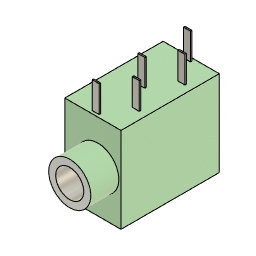
Headphone amplifier II v17 (Autodesk Fusion 360 archive; units mm, degrees)
design "Jack"
Autodesk Fusion 360 part; units mm, degrees
sketch "Sketch1" plane through (0, 0, 0) normal (0, 0, 1) x (1, 0, 0)
  line L0 (4, -7) -> (-4, -7)
  line L1 (-4, -7) -> (-4, 7)
  line L2 (-4, 7) -> (4, 7)
  line L3 (4, 7) -> (4, -7)
  line L4 (4, -7) -> (-4, 7) construction
  line L5 (-4, -7) -> (4, 7) construction
  line L6 (0.5, -0.1) -> (-0.5, -0.1)
  line L7 (-0.5, -0.1) -> (-0.5, 0.1)
  line L8 (-0.5, 0.1) -> (0.5, 0.1)
  line L9 (0.5, 0.1) -> (0.5, -0.1)
  line L10 (0.5, -0.1) -> (-0.5, 0.1) construction
  line L11 (-0.5, -0.1) -> (0.5, 0.1) construction
  line L12 (0.5, -6.6) -> (-0.5, -6.6)
  line L13 (-0.5, -6.6) -> (-0.5, -6.4)
  line L14 (0.5, -6.4) -> (0.5, -6.6)
  line L15 (-0.5, -6.4) -> (0.5, -6.4)
  line L16 (2.959, -3.35) -> (1.959, -3.35)
  line L17 (1.959, -3.35) -> (1.959, -3.15)
  line L18 (2.959, -3.15) -> (2.959, -3.35)
  line L19 (1.959, -3.15) -> (2.959, -3.15)
  line L20 (2.959, 3.15) -> (1.959, 3.15)
  line L21 (1.959, 3.15) -> (1.959, 3.35)
  line L22 (2.959, 3.35) -> (2.959, 3.15)
  line L23 (1.959, 3.35) -> (2.959, 3.35)
  line L24 (0.5, 6.4) -> (-0.5, 6.4)
  line L25 (-0.5, 6.4) -> (-0.5, 6.6)
  line L26 (0.5, 6.6) -> (0.5, 6.4)
  line L27 (-0.5, 6.6) -> (0.5, 6.6)
  dimension "d61" = 8
  dimension "d62" = 14
  dimension "d63" = 1
  dimension "d64" = 0.2
  dimension "d67" = 2.459
  dimension "d68" = 6.5
  constraint horizontal L0
  constraint perpendicular L0 L1
  constraint parallel L0 L2
  constraint parallel L1 L3
  constraint coincident L4 origin
  constraint coincident L5 origin
  constraint horizontal L6
  constraint perpendicular L6 L7
  constraint parallel L6 L8
  constraint parallel L7 L9
  constraint coincident L10 origin
  constraint coincident L11 origin
  measures "d61" distance of L1.end L2.end
  measures "d62" distance of L0.end L1.end
  measures "d63" distance of L7.end L8.end
  measures "d64" distance of L6.end L7.end
extrude "Extrude1" add sketch "Sketch1" along normal blind 16 contours L6 L7 L8 L9 | L12 L13 L14 L15 | L16 L17 L18 L19 | L20 L21 L22 L23 | L24 L25 L26 L27 makes body 1 at (0.1667, -0.1, 5.3333) makes body 2 at (2.6257, 3.15, 5.3333) makes body 3 at (2.6257, -3.35, 5.3333) makes body 4 at (0.1667, 6.4, 5.3333) makes body 5 at (0.1667, -6.6, 5.3333)
extrude "Extrude2" add sketch "Sketch1" along normal blind 12.2 bodies 1 2 3 4 5
sketch "Sketch2" plane through (0, -7, 0) normal (0, -1, 0) x (1, 0, 0)
  line L0 (-4, 0) -> (4, 0)
  line L1 (4, 0) -> (4, 12.2)
  line L2 (4, 12.2) -> (-4, 12.2)
  line L3 (-4, 12.2) -> (-4, 0)
  circle A0 centre (0.7, 6) radius 3
  circle A1 centre (0.7, 6) radius 2
  line L4 (4, 0) -> (-4, 0)
  dimension "d73" = 6
  dimension "d74" = -1
  dimension "d76" = 3.3
  dimension "d78" = 6
  measures "d73" diameter of A0
  measures "d76" distance of L1 A0.centre
  measures "d78" distance of A0.centre L4
extrude "Extrude3" add sketch "Sketch2" along normal blind 4 contours A0 bodies 1
extrude "Extrude4" cut sketch "Sketch2" against normal blind 12 contours A1 bodies 1
named bodies: "JackFem"

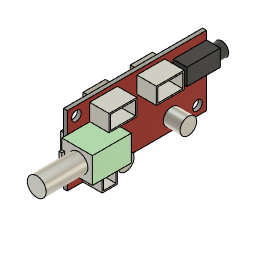
design "Amplifier"
Autodesk Fusion 360 part; units mm, degrees
sketch "Sketch1" plane through (0, 0, 0) normal (0, 0, 1) x (1, 0, 0)
  line L0 (12.5, -25) -> (-12.5, -25)
  line L1 (-12.5, -25) -> (-12.5, 25)
  line L2 (-12.5, 25) -> (12.5, 25)
  line L3 (12.5, 25) -> (12.5, -25)
  line L4 (12.5, -25) -> (-12.5, 25) construction
  line L5 (-12.5, -25) -> (12.5, 25) construction
  circle A0 centre (9.25, 21.75) radius 1.75
  circle A1 centre (-9.25, -21.75) radius 1.75
  line L6 (4.3, -27) -> (-5, -27)
  line L7 (-5, -27) -> (-5, -13)
  line L8 (-5, -13) -> (4.3, -13)
  line L9 (4.3, -13) -> (4.3, -27)
  line L10 (4.3, -27) -> (-5, -13) construction
  line L11 (-5, -27) -> (4.3, -13) construction
  line L12 (-3.5, 13) -> (-9.5, 13)
  line L13 (-9.5, 13) -> (-9.5, 25)
  line L14 (-9.5, 25) -> (-3.5, 25)
  line L15 (-3.5, 25) -> (-3.5, 13)
  line L16 (-3.5, 13) -> (-9.5, 25) construction
  line L17 (-9.5, 13) -> (-3.5, 25) construction
  line L18 (-11.1, -7) -> (-5.1, -7)
  line L19 (-5.1, -7) -> (-5.1, -17)
  line L20 (-5.1, -17) -> (-11.1, -17)
  line L21 (-11.1, -17) -> (-11.1, -7)
  line L22 (-11.1, -7) -> (-5.1, -17) construction
  line L23 (-5.1, -7) -> (-11.1, -17) construction
  line L24 (-10.6, -7.5) -> (-5.6, -7.5)
  line L25 (-5.6, -7.5) -> (-5.6, -16.5)
  line L26 (-5.6, -16.5) -> (-10.6, -16.5)
  line L27 (-10.6, -16.5) -> (-10.6, -7.5)
  line L28 (-11.1, 0) -> (-11.1, 10)
  line L29 (-11.1, 10) -> (-5.1, 10)
  line L30 (-5.1, 10) -> (-5.1, 0)
  line L31 (-5.1, 0) -> (-11.1, 0)
  line L32 (-10.6, 0.5) -> (-10.6, 9.5)
  line L33 (-10.6, 9.5) -> (-5.6, 9.5)
  line L34 (-5.6, 0.5) -> (-10.6, 0.5)
  line L35 (-5.6, 9.5) -> (-5.6, 0.5)
  circle A2 centre (8, 12.5) radius 3
  circle A3 centre (8, -10) radius 3
  line L36 (4.4, -14) -> (12.4, -14)
  line L37 (12.4, -14) -> (12.4, -19.5)
  line L38 (12.4, -19.5) -> (4.4, -19.5)
  line L39 (4.4, -19.5) -> (4.4, -14)
  line L40 (4.4, -14) -> (12.4, -19.5) construction
  line L41 (12.4, -14) -> (4.4, -19.5) construction
  line L42 (4.9, -14.5) -> (11.9, -14.5)
  line L43 (11.9, -14.5) -> (11.9, -19)
  line L44 (11.9, -19) -> (4.9, -19)
  line L45 (4.9, -19) -> (4.9, -14.5)
  point P0 (-0.35, -20)
  point P1 (-6.5, 19)
  point P2 (-8.1, -12)
  point P3 (8.4, -16.75)
  dimension "d1" = 25
  dimension "d2" = 50
  dimension "d3" = 3.5
  dimension "d4" = 3.25
  dimension "d5" = 3.25
  dimension "d6" = 3.25
  dimension "d7" = 3.25
  dimension "d8" = 9.3
  dimension "d9" = 14
  dimension "d10" = 7.5
  dimension "d11" = 2
  dimension "d12" = 12
  dimension "d13" = 6
  dimension "d15" = 3
  dimension "d30" = 6
  dimension "d31" = 10
  dimension "d32" = 0.5
  dimension "d33" = 0.5
  dimension "d34" = 6
  dimension "d35" = 10
  dimension "d37" = 8
  dimension "d38" = 7
  dimension "d39" = 1.4
  dimension "d40" = 6
  dimension "d41" = 12.5
  dimension "d42" = 35
  dimension "d43" = 4.5
  dimension "d44" = 8
  dimension "d45" = 5.5
  dimension "d46" = 0.5
  dimension "d47" = 0.1
  dimension "d48" = 5.5
  constraint horizontal L0
  constraint perpendicular L0 L1
  constraint parallel L0 L2
  constraint parallel L1 L3
  constraint coincident L4 origin
  constraint coincident L5 origin
  constraint equal A0 A1
  constraint horizontal L6
  constraint perpendicular L6 L7
  constraint parallel L6 L8
  constraint parallel L7 L9
  constraint coincident L10 P0
  constraint coincident L11 P0
  constraint horizontal L12
  constraint perpendicular L12 L13
  constraint parallel L12 L14
  constraint parallel L13 L15
  constraint coincident L16 P1
  constraint coincident L17 P1
  constraint horizontal L18
  constraint perpendicular L18 L19
  constraint parallel L18 L20
  constraint parallel L19 L21
  constraint coincident L22 P2
  constraint coincident L23 P2
  constraint horizontal L29
  constraint perpendicular L29 L30
  constraint parallel L29 L31
  constraint parallel L28 L30
  constraint vertical L18.end L30.end
  constraint equal A2 A3
  constraint vertical A2.centre A3.centre
  constraint horizontal L36
  constraint perpendicular L36 L37
  constraint parallel L36 L38
  constraint parallel L37 L39
  constraint coincident L40 P3
  constraint coincident L41 P3
  constraint coincident L2 L13.end
  measures "d1" distance of L1.end L2.end
  measures "d2" distance of L0.end L1.end
  measures "d3" diameter of A0
  measures "d4" distance of L2 A0.centre
  measures "d5" distance of L3 A0.centre
  measures "d6" distance of L1 A1.centre
  measures "d7" distance of L0 A1.centre
  measures "d8" distance of L7.end L8.end
  measures "d9" distance of L6.end L7.end
  measures "d10" distance of L1 L7
  measures "d11" distance of L0 L6
  measures "d12" distance of L12.start L14.end
  measures "d13" distance of L12.start L12.end
  measures "d15" distance of L1 L13
  measures "d30" distance of L19.end L20.end
  measures "d31" distance of L18.end L19.end
  measures "d34" distance of L30.end L28.start
  measures "d35" distance of L29.end L30.end
  measures "d37" distance of L0 L20
  measures "d38" distance of L18 L31
  measures "d39" distance of L1 L21
  measures "d40" diameter of A2
  measures "d41" distance of L2 A2.centre
  measures "d42" distance of L2 A3.centre
  measures "d43" distance of L3 A2.centre
  measures "d44" distance of L37.end L38.end
  measures "d45" distance of L36.end L37.end
  measures "d47" distance of L3 L37
  measures "d48" distance of L0 L38
extrude "Extrude1" add sketch "Sketch1" against normal blind 1.4 contours L0 L1 L2 L3 L7 L8 L9 L12 L13 L15 | L0 L7 L8 L9 | L2 L12 L13 L14 L15 | L18 L19 L20 L21 | L24 L25 L26 L27 | L28 L29 L30 L31 | L32 L33 L34 L35 | A2 | A3 | L36 L37 L38 L39 | L42 L43 L44 L45
sketch "Sketch5" plane through (0, 0, -1.4) normal (0, 0, -1) x (1, 0, 0)
  circle A0 centre (9.25, -21.75) radius 1.75
  circle A1 centre (-9.25, 21.75) radius 1.75
  line L0 (-12.5, -25) -> (12.5, -25)
  line L1 (12.5, -25) -> (12.5, 25)
  line L2 (12.5, 25) -> (-12.5, 25)
  line L3 (-12.5, 25) -> (-12.5, -25)
  line L4 (-7, 8) -> (-12, 8)
  line L5 (-12, 8) -> (-12, 16)
  line L6 (-12, 16) -> (-7, 16)
  line L7 (-7, 16) -> (-7, 8)
  line L8 (-7, 8) -> (-12, 16) construction
  line L9 (-12, 8) -> (-7, 16) construction
  line L10 (-7, -1) -> (-7, -9)
  line L11 (-7, -9) -> (-12, -9)
  line L12 (-12, -9) -> (-12, -1)
  line L13 (-12, -1) -> (-7, -1)
  line L14 (4, 19) -> (-4, 19)
  line L15 (-4, 19) -> (-4, 24)
  line L16 (-4, 24) -> (4, 24)
  line L17 (4, 24) -> (4, 19)
  line L18 (4, 12) -> (-4, 12)
  line L19 (-4, 12) -> (-4, 17)
  line L20 (-4, 17) -> (4, 17)
  line L21 (4, 17) -> (4, 12)
  line L22 (11.5, 17) -> (5.5, 17)
  line L23 (5.5, 17) -> (5.5, 20)
  line L24 (5.5, 20) -> (11.5, 20)
  line L25 (11.5, 20) -> (11.5, 17)
  line L26 (11.5, 17) -> (5.5, 20) construction
  line L27 (5.5, 17) -> (11.5, 20) construction
  line L28 (4, 24) -> (-4, 19) construction
  line L29 (-4, 24) -> (4, 19) construction
  point P0 (-9.5, 12)
  point P1 (8.5, 18.5)
  point P2 (0, 21.5)
  dimension "d100" = 5
  dimension "d101" = 8
  dimension "d104" = 5
  dimension "d105" = 8
  dimension "d106" = 5
  dimension "d107" = 8
  dimension "d108" = 5
  dimension "d109" = 8
  dimension "d110" = 6
  dimension "d111" = 3
  dimension "d112" = 13
  dimension "d113" = 26
  dimension "d114" = 3
  dimension "d115" = 12.5
  dimension "d116" = 1
  dimension "d117" = 8
  dimension "d118" = 5
  dimension "d119" = 1
  constraint horizontal L4
  constraint perpendicular L4 L5
  constraint parallel L4 L6
  constraint parallel L5 L7
  constraint coincident L8 P0
  constraint coincident L9 P0
  constraint horizontal L11
  constraint perpendicular L11 L12
  constraint parallel L11 L13
  constraint parallel L10 L12
  constraint perpendicular L15 L16
  constraint parallel L15 L17
  constraint parallel L14 L16
  constraint perpendicular L19 L20
  constraint parallel L19 L21
  constraint parallel L18 L20
  constraint horizontal L22
  constraint perpendicular L22 L23
  constraint parallel L22 L24
  constraint parallel L23 L25
  constraint coincident L26 P1
  constraint coincident L27 P1
  constraint vertical L4.end L12.end
  constraint vertical L14.end L19.end
  constraint parallel L17 L21
  constraint midpoint L28 P2
  measures "d100" distance of L5.end L6.end
  measures "d101" distance of L4.end L5.end
  measures "d104" distance of L12.end L10.start
  measures "d105" distance of L12.end L11.end
  measures "d106" distance of L16.end L14.start
  measures "d107" distance of L16.end L15.end
  measures "d108" distance of L20.end L18.start
  measures "d109" distance of L20.end L19.end
  measures "d110" distance of L23.end L24.end
  measures "d111" distance of L22.end L23.end
  measures "d112" distance of L2 P0
  measures "d113" distance of L2 L13
  measures "d114" distance of L3 P0
  measures "d115" distance of L3 P2
  measures "d116" distance of L2 L16
  measures "d117" distance of L2 L20
  measures "d118" distance of L2 L24
  measures "d119" distance of L1 L25
extrude "Extrude11" add sketch "Sketch5" along normal blind 2 contours L4 L5 L6 L7 | L10 L11 L12 L13 | L14 L15 L16 L17 | L18 L19 L20 L21 | L22 L23 L24 L25
extrude "Extrude2" add sketch "Sketch1" along normal blind 5 contours L2 L12 L13 L14 L15
extrude "Extrude10" add sketch "Sketch1" along normal blind 7 contours L36 L37 L38 L39
sketch "Sketch3" plane through (0, 25, 0) normal (0, 1, 0) x (-1, 0, 0)
  line L0 (12.5, 0) -> (9.5, 0)
  line L1 (9.5, 0) -> (9.5, 5)
  line L2 (9.5, 5) -> (3.5, 5)
  line L3 (3.5, 5) -> (3.5, 0)
  line L4 (3.5, 0) -> (-12.5, 0)
  line L5 (-12.5, 0) -> (-12.5, -1.4)
  line L6 (-12.5, -1.4) -> (12.5, -1.4)
  line L7 (12.5, -1.4) -> (12.5, 0)
sketch "Sketch4" plane through (0, 25, 1.8) normal (0, 1, 0) x (-1, 0, 0)
  line L0 (9.5, 3.2) -> (3.5, 3.2)
  line L1 (3.5, 3.2) -> (3.5, -1.8)
  circle A0 centre (6.5, 0.7) radius 2.5
  circle A1 centre (6.5, 0.7) radius 2
  point P0 (6.5, 3.2)
  point P1 (3.5, 0.7)
  dimension "d53" = 5
  dimension "d54" = -0.5
  constraint midpoint L0 P0
  constraint midpoint L1 P1
  constraint vertical P0 A0.centre
  constraint horizontal P1 A0.centre
  measures "d53" diameter of A0
extrude "Extrude8" add sketch "Sketch4" along normal blind 3
extrude "Extrude9" cut sketch "Sketch4" against normal blind 10 contours A1
extrude "Extrude3" add sketch "Sketch1" along normal blind 11 contours L0 L6 L7 L9 | L0 L7 L8 L9
sketch "Sketch2" plane through (0, -27, 0) normal (0, -1, 0) x (1, 0, 0)
  line L0 (-5, 0) -> (4.3, 0)
  line L1 (4.3, 0) -> (4.3, 11)
  line L2 (4.3, 11) -> (-5, 11)
  line L3 (-5, 11) -> (-5, 0)
  circle A0 centre (-0.35, 6) radius 3.4
  line L4 (0.65, 0) -> (-1.35, 0)
  line L5 (-1.35, 0) -> (-1.35, 1)
  line L6 (-1.35, 1) -> (0.65, 1)
  line L7 (0.65, 1) -> (0.65, 0)
  line L8 (0.65, 0) -> (-1.35, 1) construction
  line L9 (-1.35, 0) -> (0.65, 1) construction
  point P0 (-0.35, 11)
  point P1 (-0.35, 0.5)
  point P2 (-0.35, 0)
  dimension "d22" = 6.8
  dimension "d23" = 5
  dimension "d26" = 2
  dimension "d27" = 1
  constraint midpoint L2 P0
  constraint vertical A0.centre P0
  constraint horizontal L4
  constraint perpendicular L4 L5
  constraint parallel L4 L6
  constraint parallel L5 L7
  constraint coincident L8 P1
  constraint coincident L9 P1
  constraint vertical A0.centre P1
  constraint coincident L4 P2
  measures "d22" diameter of A0
  measures "d23" distance of L2 A0.centre
  measures "d26" distance of L5.end L6.end
  measures "d27" distance of L4.end L5.end
extrude "Extrude4" add sketch "Sketch2" along normal blind 15 contours A0
extrude "Extrude5" add sketch "Sketch2" along normal blind 1 contours L0 L4 L5 L6 L7
extrude "Extrude6" add sketch "Sketch1" along normal blind 6 contours A2 | A3
extrude "Extrude7" add sketch "Sketch1" along normal blind 7 contours L18 L19 L20 L21 | L28 L29 L30 L31
move_body "Move1" bodies 1 to x (0, 0, -1) y (0, 1, 0) z (1, 0, 0) at (-9.1, 0, -15.9)
equation "d4 = d3 / 2 + 1.5 mm"
equation "d5 = d4"
equation "d6 = d4"
equation "d7 = d4"
named bodies: "Amplifier"
